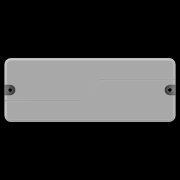
# Autodesk Inventor part: fishman-modern8
Saved by Autodesk Inventor 2020 (Build 240168000, 168)
## iProperties
Created: 2020-01-01
Part Number: fishman-modern8
Material: Generic
Document SubType Name: Modeling
Designer: valer
Density: 1 g/cm^3
Appearance: Default
Author: valer
Autodesk Inventor part; units mm, degrees
ref_plane "YZ Plane" through (0, 0, 0) normal (1, 0, 0) x (0, 1, 0)
ref_plane "XZ Plane" through (0, 0, 0) normal (0, 1, 0) x (-1, 0, 0)
ref_plane "XY Plane" through (0, 0, 0) normal (0, 0, 1) x (1, 0, 0)
sketch "FishmanModern8" plane through (0, 0, 0) normal (0, 0, 1) x (1, 0, 0)
  line L0 (-50.9143, 0) -> (50.9143, 0) construction
  line L1 (0, 18.9484) -> (0, -18.9484) construction
  line L2 (-50.9143, 18.9484) -> (50.9143, 18.9484)
  line L3 (50.9143, 18.9484) -> (50.9143, -18.9484)
  line L4 (50.9143, -18.9484) -> (-50.9143, -18.9484)
  line L5 (-50.9143, -18.9484) -> (-50.9143, 18.9484)
  circle A0 centre (-47.625, 0) radius 1.27
  circle A1 centre (47.625, 0) radius 1.27
  line L6 (-3.3542, -4.7903) -> (3.3542, 4.7903)
  line L7 (-6.3503, -6.35) -> (-50.9143, -6.35)
  line L8 (6.3503, 6.35) -> (50.9143, 6.35)
  circle A2 centre (-47.625, 0) radius 3.175
  circle A3 centre (47.625, 0) radius 3.175
  line L9 (-50.9143, 3.175) -> (-47.625, 3.175)
  line L10 (-50.9143, -3.175) -> (-47.625, -3.175)
  line L11 (47.625, 3.175) -> (50.9143, 3.175)
  line L12 (47.625, -3.175) -> (50.9143, -3.175)
  arc A4 (6.3503, 6.35) -> (3.3542, 4.7903) centre (6.3503, 2.6924) ccw
  arc A5 (-6.3503, -6.35) -> (-3.3542, -4.7903) centre (-6.3503, -2.6924) ccw
  line L13 (50.9143, 6.731) -> (6.3503, 6.731)
  arc A6 (6.3503, 6.731) -> (3.0421, 5.0088) centre (6.3503, 2.6924) ccw
  line L14 (3.0421, 5.0088) -> (-3.6663, -4.5718)
  arc A7 (-6.3503, -5.969) -> (-3.6663, -4.5718) centre (-6.3503, -2.6924) ccw
  line L15 (-6.3503, -5.969) -> (-50.9143, -5.969)
  line L16 (50.9143, 5.969) -> (6.3503, 5.969)
  arc A8 (6.3503, 5.969) -> (3.6663, 4.5718) centre (6.3503, 2.6924) ccw
  line L17 (3.6663, 4.5718) -> (-3.0421, -5.0088)
  arc A9 (-6.3503, -6.731) -> (-3.0421, -5.0088) centre (-6.3503, -2.6924) ccw
  line L18 (-6.3503, -6.731) -> (-50.9143, -6.731)
  line L19 (-50.9143, -5.969) -> (-50.9143, -6.731)
  line L20 (50.9143, 6.731) -> (50.9143, 5.969)
  point P0 (0, 0)
  point P1 (0, 0)
  dimension "d72" = 101.8286
  dimension "d73" = 37.8968
  dimension "d74" = 2.54
  dimension "d75" = 95.25
  dimension "d76" = 47.625
  dimension "d77" = 47.625
  dimension "d78" = 55
  dimension "d79" = 6.35
  dimension "d80" = 6.35
  dimension "d81" = 6.35
  dimension "d85" = 3.6576
  dimension "d86" = 0.381
  dimension "d87" = 0.381
  constraints: 42 end point, 16 point on circle, 10 centre point, 8 tangent, 7 horizontal, 7 point on line, 5 midpoint, 3 coincident, 3 equal radius, 3 parallel, 2 perpendicular, 2 vertical, 8 other
  measures "d72" distance of L0.start L0.end
  measures "d73" distance of L1.start L1.end
  measures "d74" diameter of A0
  measures "d75" distance of A1.centre A0.centre
  measures "d76" distance from line of L1 A0.centre
  measures "d77" distance from line of A1.centre L1
  measures "d78" angle of L6 L0
  measures "d79" distance between parallel lines of L0 L7
  measures "d80" distance between parallel lines of L0 L8
  measures "d81" diameter of A2
  measures "d85" radius of A4
  measures "d86" distance between parallel lines of L8 L13
  measures "d87" distance between parallel lines of L8 L16
extrude "FishmanModern8Feature" add sketch "FishmanModern8" against normal blind 18.0086 contours L2 L3 L13 A6 L14 A7 L15 L5 L10 A2 L9 | L9 A2 L10 L5 | L3 L8 A4 L6 A5 L7 L5 L15 A7 L14 A6 L13 | A2 | L3 L16 A8 L17 A9 L18 L5 L7 A5 L6 A4 L8 | L3 L11 A3 L12 L4 L5 L18 A9 L17 A8 L16 | L3 L12 A3 L11 | A3 | A0 | A1
fillet "FishmanModern8FilletsFeature" radius 3.6576 4 edges at (-50.9143, 18.9484, -9.0043) (-50.9143, -18.9484, -9.0043) (50.9143, 18.9484, -9.0043) (50.9143, -18.9484, -9.0043)
extrude "FishmanModern8IndentFeature" cut sketch "FishmanModern8" against normal blind 1.27 contours L3 L8 A4 L6 A5 L7 L5 L15 A7 L14 A6 L13 | L3 L16 A8 L17 A9 L18 L5 L7 A5 L6 A4 L8
extrude "FishmanModern8MountsFeature" cut sketch "FishmanModern8" against normal through all contours A0 | A1
extrude "FishmanModern8CountersinksFeature" cut sketch "FishmanModern8" against normal blind 6.35 contours L9 A2 L10 L5 | A2 | L3 L12 A3 L11 | A3 | A1
chamfer "FishmanModern8ChamferFeature" distance 1.27 angle 45 12 edges at (0, 18.9484, 0) (-49.843, 17.8771, 0) (-50.9143, 9.2329, 0) (49.843, 17.8771, 0) (50.9143, 11.0109, 0) (0, -18.9484, 0) (49.843, -17.8771, 0) (50.9143, -9.2329, 0) (-49.843, -17.8771, 0) (-50.9143, -11.0109, 0) (-50.9143, -4.572, 0) (50.9143, 4.572, 0)
equation "\"d76\" = d77"
body "Solid1"
